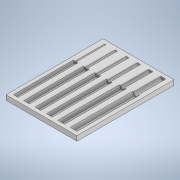
# Autodesk Inventor part: punchTray
Saved by Autodesk Inventor 2020.2 (Build 242310000, 310)
## iProperties
Created: 2019-12-07
Part Number: punchTray
Material: Generic
Document SubType Name: Modeling
Designer: robst
Density: 1 g/cm^3
Appearance: Default
Author: robst
Autodesk Inventor part; units mm, degrees
ref_plane "YZ Plane" through (0, 0, 0) normal (1, 0, 0) x (0, 1, 0)
ref_plane "XZ Plane" through (0, 0, 0) normal (0, 1, 0) x (-1, 0, 0)
ref_plane "XY Plane" through (0, 0, 0) normal (0, 0, 1) x (1, 0, 0)
sketch "Sketch3" plane through (0, 0, 0) normal (0, 0, 1) x (1, 0, 0)
  line L0 (-60.4011, -4.0957) -> (60.4011, -4.0957)
  line L1 (60.4011, -4.0957) -> (60.4011, 4.0957)
  line L2 (60.4011, 4.0957) -> (-60.4011, 4.0957)
  line L3 (-60.4011, 4.0957) -> (-60.4011, -4.0957)
  line L4 (-60.4011, -4.0957) -> (60.4011, 4.0957) construction
  line L5 (60.4011, -4.0957) -> (-60.4011, 4.0957) construction
  line L6 (54.0511, 4.0957) -> (51.1548, -0.9208)
  line L7 (51.1548, -0.9208) -> (45.3623, -0.9208)
  line L8 (45.3623, -0.9208) -> (42.466, 4.0957)
  line L9 (42.466, 4.0957) -> (45.3623, 9.1122)
  line L10 (45.3623, 9.1122) -> (51.1548, 9.1123)
  line L11 (51.1548, 9.1123) -> (54.0511, 4.0957)
  line L12 (32.941, 4.0957) -> (30.0447, -0.9208)
  line L13 (30.0447, -0.9208) -> (24.2522, -0.9208)
  line L14 (24.2522, -0.9208) -> (21.3559, 4.0957)
  line L15 (21.3559, 4.0957) -> (24.2522, 9.1122)
  line L16 (24.2522, 9.1122) -> (30.0447, 9.1122)
  line L17 (30.0447, 9.1122) -> (32.941, 4.0957)
  line L18 (0, 0) -> (0, 4.0957) construction
  line L19 (11.8309, 4.0957) -> (9.3745, -0.1588)
  line L20 (9.3745, -0.1588) -> (4.4619, -0.1588)
  line L21 (4.4619, -0.1588) -> (2.0055, 4.0957)
  line L22 (2.0055, 4.0957) -> (4.4619, 8.3502)
  line L23 (4.4619, 8.3502) -> (9.3745, 8.3502)
  line L24 (9.3745, 8.3502) -> (11.8309, 4.0957)
  line L25 (-7.5195, 4.0957) -> (-9.9758, -0.1588)
  line L26 (-9.9758, -0.1588) -> (-14.8885, -0.1588)
  line L27 (-14.8885, -0.1588) -> (-17.3448, 4.0957)
  line L28 (-17.3448, 4.0957) -> (-14.8885, 8.3502)
  line L29 (-14.8885, 8.3502) -> (-9.9758, 8.3502)
  line L30 (-9.9758, 8.3502) -> (-7.5195, 4.0957)
  line L31 (-26.8698, 4.0957) -> (-29.3041, -0.1207)
  line L32 (-29.3041, -0.1207) -> (-34.1728, -0.1206)
  line L33 (-34.1728, -0.1206) -> (-36.6072, 4.0958)
  line L34 (-36.6072, 4.0958) -> (-34.1728, 8.3121)
  line L35 (-34.1728, 8.3121) -> (-29.3041, 8.3121)
  line L36 (-29.3041, 8.3121) -> (-26.8698, 4.0957)
  line L37 (-46.1322, 4.0957) -> (-48.1119, 0.6667)
  line L38 (-48.1119, 0.6667) -> (-52.0714, 0.6667)
  line L39 (-52.0714, 0.6667) -> (-54.0511, 4.0957)
  line L40 (-54.0511, 4.0957) -> (-52.0714, 7.5247)
  line L41 (-52.0714, 7.5247) -> (-48.1119, 7.5248)
  line L42 (-48.1119, 7.5248) -> (-46.1322, 4.0957)
  point P0 (48.2585, 4.0957)
  point P1 (27.1484, 4.0957)
  point P2 (42.466, 4.0957)
  point P3 (21.3559, 4.0957)
  point P4 (6.9182, 4.0957)
  point P5 (-12.4321, 4.0957)
  point P6 (-31.7385, 4.0957)
  point P7 (-50.0916, 4.0957)
  point P8 (2.0055, 4.0957)
  point P9 (-17.3448, 4.0957)
  point P10 (-36.6072, 4.0957)
  point P11 (-54.0511, 4.0957)
  dimension "d7" = 10.033
  dimension "d8" = 10.033
  dimension "d13" = 6.35
  dimension "d14" = 9.525
  dimension "d15" = 8.509
  dimension "d16" = 9.525
  dimension "d17" = 8.509
  dimension "d18" = 9.525
  dimension "d19" = 8.4328
  dimension "d20" = 9.525
  dimension "d21" = 9.525
  dimension "d22" = 6.858
  dimension "d23" = 6.35
  dimension "d24" = 3.175
  constraints: 84 end point, 2 horizontal, 2 midpoint, 1 parallel, 1 perpendicular, 94 other
  measures "d7" distance between parallel lines of L7 L10
  measures "d8" distance between parallel lines of L13 L16
  measures "d13" distance of L6.start L1.end
  measures "d14" distance of L8.end L12.start
  measures "d15" distance between parallel lines of L20 L23
  measures "d16" distance of L14.end L19.start
  measures "d17" distance between parallel lines of L26 L29
  measures "d18" distance of L21.end L25.start
  measures "d19" distance between parallel lines of L32 L35
  measures "d20" distance of L27.end L31.start
  measures "d21" distance of L33.end L37.start
  measures "d22" distance between parallel lines of L38 L41
  measures "d23" distance from line of L39.end L3
  measures "d24" distance between parallel lines of L0 L7
extrude "Extrusion3" add sketch "Sketch3" against normal blind 152.4 contours L3 L2 L39 L38 L37 L33 L32 L31 L27 L26 L25 L21 L20 L19 L14 L13 L12 L8 L7 L6 L1 L0
sketch "Sketch4" plane through (0, 0, 0) normal (0, 0, 1) x (1, 0, 0)
  line L0 (60.4011, -4.0957) -> (-60.4011, -4.0957) projected
  line L1 (60.4011, 4.0957) -> (60.4011, -4.0957) projected
  line L2 (-60.4011, -4.0957) -> (60.4011, -4.0957)
  line L3 (60.4011, -4.0957) -> (60.4011, 4.0957)
  line L4 (60.4011, 4.0957) -> (-60.4011, 4.0957)
  line L5 (-60.4011, 4.0957) -> (-60.4011, -4.0957)
  point P0 (0, 0)
  constraints: 8 end point, 2 parallel, 1 horizontal, 1 perpendicular
extrude "Extrusion4" add sketch "Sketch4" along normal blind 6.35
sketch "Sketch6" plane through (0, 0, -152.4) normal (0, 0, -1) x (-1, 0, 0)
  line L0 (-45.3623, -0.9208) -> (-51.1548, -0.9208) construction
  line L1 (-48.2585, -0.9208) -> (-48.2585, 4.0957) construction
  line L2 (-60.4011, 4.0957) -> (60.4011, 4.0957) construction
  arc A0 (-52.4813, 4.0957) -> (-44.0358, 4.0957) centre (-48.2585, 4.0957) ccw
  line L3 (-42.466, 4.0957) -> (-45.3623, -0.9208)
  line L4 (-45.3623, -0.9208) -> (-51.1548, -0.9208)
  line L5 (-51.1548, -0.9208) -> (-54.0511, 4.0957)
  line L6 (-54.0511, 4.0957) -> (-52.4813, 4.0957)
  line L7 (-42.466, 4.0957) -> (-44.0358, 4.0957)
  point P0 (0, 0)
  dimension "d31" = 8.4455
  constraints: 12 end point, 3 point on line, 2 coincident, 2 point on circle, 1 centre point, 1 midpoint, 1 vertical, 6 other
  measures "d31" diameter of A0
extrude "5_16_punch" add sketch "Sketch6" against normal blind 46.355
sketch "Sketch7" plane through (0, 0, -152.4) normal (0, 0, -1) x (-1, 0, 0)
  line L0 (-32.941, 4.0957) -> (-21.3559, 4.0957) projected
  line L1 (-21.3559, 4.0957) -> (-24.2522, -0.9208)
  line L2 (-24.2522, -0.9208) -> (-30.0447, -0.9208)
  line L3 (-30.0447, -0.9208) -> (-32.941, 4.0957)
  arc A0 (-30.5774, 4.0957) -> (-23.7194, 4.0957) centre (-27.1484, 4.0957) ccw
  line L4 (-32.941, 4.0957) -> (-30.5774, 4.0957)
  line L5 (-11.8309, 4.0957) -> (-21.3559, 4.0957) projected
  line L6 (-21.3559, 4.0957) -> (-23.7194, 4.0957)
  point P0 (0, 0)
  dimension "d34" = 6.858
  constraints: 10 end point, 2 point on circle, 2 point on line, 1 centre point, 1 coincident, 1 midpoint, 6 other
  measures "d34" diameter of A0
extrude "1_4_punch" add sketch "Sketch7" against normal blind 47.625 contours L0 A0 L1 L2 L3
sketch "Sketch8" plane through (0, 0, -152.4) normal (0, 0, -1) x (-1, 0, 0)
  line L0 (-11.8309, 4.0957) -> (-2.0055, 4.0957) projected
  line L1 (-2.0055, 4.0957) -> (-4.4619, -0.1588)
  line L2 (-4.4619, -0.1588) -> (-9.3745, -0.1588)
  line L3 (-9.3745, -0.1588) -> (-11.8309, 4.0957)
  arc A0 (-9.5535, 4.0957) -> (-4.283, 4.0957) centre (-6.9182, 4.0957) ccw
  line L4 (-11.8309, 4.0957) -> (-9.3745, -0.1588) projected
  line L5 (-11.8309, 4.0957) -> (-9.5535, 4.0957)
  line L6 (-2.0055, 4.0957) -> (-4.283, 4.0957)
  point P0 (0, 0)
  dimension "d37" = 5.2705
  constraints: 10 end point, 2 point on circle, 2 point on line, 1 centre point, 1 coincident, 1 midpoint, 6 other
  measures "d37" diameter of A0
extrude "3_16_punch" add sketch "Sketch8" against normal blind 50.8 contours L0 A0 L1 L2 L3
sketch "Sketch9" plane through (0, 0, -152.4) normal (0, 0, -1) x (-1, 0, 0)
  line L0 (14.8885, -0.1588) -> (9.9758, -0.1588) construction
  line L1 (12.4321, -0.1588) -> (12.4321, 4.0957) construction
  line L2 (-60.4011, 4.0957) -> (60.4011, 4.0957) construction
  line L3 (17.3448, 4.0957) -> (14.8885, -0.1588) projected
  line L4 (17.3448, 4.0957) -> (14.8885, -0.1587)
  line L5 (14.8885, -0.1587) -> (9.9758, -0.1588)
  line L6 (9.9758, -0.1588) -> (7.5195, 4.0957)
  arc A0 (10.1938, 4.0957) -> (14.6705, 4.0957) centre (12.4321, 4.0957) ccw
  line L7 (9.9758, -0.1588) -> (7.5195, 4.0957) projected
  line L8 (7.5195, 4.0957) -> (10.1938, 4.0957)
  line L9 (26.8698, 4.0957) -> (17.3448, 4.0957) projected
  line L10 (17.3448, 4.0957) -> (14.6705, 4.0957)
  point P0 (0, 0)
  point P1 (14.8885, -0.1588)
  dimension "d40" = 4.4768
  constraints: 12 end point, 3 point on line, 2 coincident, 2 point on circle, 1 centre point, 1 midpoint, 1 vertical, 6 other
  measures "d40" diameter of A0
extrude "5_32_punch" add sketch "Sketch9" against normal blind 50.8
sketch "Sketch11" plane through (0, 0, -152.4) normal (0, 0, -1) x (-1, 0, 0)
  line L0 (26.8698, 4.0957) -> (36.6072, 4.0957) projected
  line L1 (34.1728, -0.1206) -> (36.6072, 4.0957) projected
  line L2 (36.6072, 4.0957) -> (34.1728, -0.1206)
  line L3 (34.1728, -0.1206) -> (29.3041, -0.1207)
  line L4 (29.3041, -0.1207) -> (26.8698, 4.0957)
  arc A0 (29.897, 4.0957) -> (33.58, 4.0957) centre (31.7385, 4.0957) ccw
  line L5 (26.8698, 4.0957) -> (29.3041, -0.1207) projected
  line L6 (26.8698, 4.0957) -> (29.897, 4.0957)
  line L7 (36.6072, 4.0957) -> (33.58, 4.0957)
  point P0 (0, 0)
  dimension "d44" = 3.683
  constraints: 10 end point, 2 point on circle, 2 point on line, 1 centre point, 1 coincident, 1 midpoint, 6 other
  measures "d44" diameter of A0
extrude "1_8_punch" add sketch "Sketch11" against normal blind 50.8 contours L0 A0 L1 L3 L4
sketch "Sketch12" plane through (0, 0, -152.4) normal (0, 0, -1) x (-1, 0, 0)
  line L0 (48.1119, 0.6667) -> (52.0714, 0.6667) construction
  line L1 (50.0916, 0.6667) -> (50.0916, 4.0957) construction
  line L2 (-60.4011, 4.0957) -> (60.4011, 4.0957) construction
  line L3 (52.0714, 0.6667) -> (54.0511, 4.0957) projected
  line L4 (54.0511, 4.0957) -> (52.0714, 0.6667)
  line L5 (52.0714, 0.6667) -> (48.1119, 0.6667)
  line L6 (48.1119, 0.6667) -> (46.1322, 4.0957)
  arc A0 (49.0439, 4.0957) -> (51.1394, 4.0957) centre (50.0916, 4.0957) ccw
  line L7 (46.1322, 4.0957) -> (33.58, 4.0957) projected
  line L8 (46.1322, 4.0957) -> (49.0439, 4.0957)
  line L9 (54.0511, 4.0957) -> (51.1394, 4.0957)
  point P0 (0, 0)
  dimension "d47" = 2.0955
  constraints: 12 end point, 3 point on line, 2 coincident, 2 point on circle, 1 centre point, 1 midpoint, 1 vertical, 6 other
  measures "d47" diameter of A0
extrude "1_16_punch" add sketch "Sketch12" against normal blind 50.8
sketch "Sketch5" plane through (0, 0, -152.4) normal (0, 0, -1) x (-1, 0, 0)
  line L0 (-60.4011, 4.0957) -> (-60.4011, -4.0957) projected
  line L1 (60.4011, 4.0957) -> (54.0511, 4.0957) projected
  line L2 (-60.4011, -4.0957) -> (60.4011, -4.0957)
  line L3 (60.4011, -4.0957) -> (60.4011, 4.0957)
  line L4 (60.4011, 4.0957) -> (-60.4011, 4.0957)
  line L5 (-60.4011, 4.0957) -> (-60.4011, -4.0957)
  point P0 (0, 0)
  constraints: 8 end point, 2 parallel, 1 horizontal, 1 perpendicular
extrude "Extrusion5" add sketch "Sketch5" along normal blind 6.35
equation "\"d14\" = gapBetweenParts"
equation "\"d16\" = gapBetweenParts"
equation "\"d18\" = gapBetweenParts"
equation "\"d20\" = gapBetweenParts"
equation "\"d21\" = gapBetweenParts"
equation "\"gapBetweenParts\" = 9.525"
body "Solid3"
